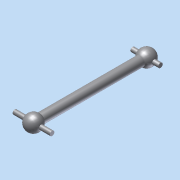
# Autodesk Inventor part: Tie Rod
Saved by Autodesk Inventor 2011 SP1 (Build 150282100, 282)
## iProperties
Created: 2011-09-20
Part Number: Tie Rod
Document SubType Name: Modeling
Designer: dgitz
Density: 1 g/cm^3
Author: dgitz
Autodesk Inventor part; units mm, degrees
ref_plane "XZ Plane" through (0, 0, 0) normal (0, 1, 0) x (-1, 0, 0)
sketch "Sketch1" plane through (0, 0, 0) normal (0, 0, 1) x (1, 0, 0)
  circle A0 centre (0, 0) radius 2.032
  dimension "d0" = 4.064
  constraints: 1 centre point, 1 coincident
  measures "d0" diameter of A0
extrude "Extrusion1" add sketch "Sketch1" along normal mid plane 42.926
sketch "Sketch2" plane through (0, 0, 0) normal (0, 1, 0) x (-1, 0, 0)
  arc A0 (2.032, 21.463) -> (0, 27.6541) centre (0, 24.2251) ccw
  line L0 (0, 21.463) -> (2.032, 21.463)
  line L1 (2.032, -21.463) -> (-2.032, -21.463) projected
  line L2 (-2.032, -21.463) -> (-2.032, 21.463) projected
  line L3 (-2.032, 21.463) -> (2.032, 21.463) projected
  line L4 (2.032, 21.463) -> (2.032, -21.463) projected
  line L5 (12.7779, 0) -> (0, 0) construction
  arc A1 (-2.032, -21.463) -> (0, -27.6541) centre (0, -24.2251) ccw
  line L6 (-2.032, -21.463) -> (0, -21.463)
  line L7 (0, 21.463) -> (0, 27.6541)
  line L8 (2.032, -21.463) -> (-2.032, -21.463) projected
  line L9 (0, -27.6541) -> (0, -21.463)
  point P0 (0, -24.5585)
  dimension "d3" = 6.858
  constraints: 10 end point, 4 point on circle, 2 centre point, 2 horizontal, 2 midpoint, 2 symmetric about line, 2 vertical, 1 point on line, 1 other
  measures "d3" diameter of A0
revolve "Revolution1" add sketch "Sketch2" angle 360 about axis through (0, 0, 21.463) along (0, 0, 1) contours L0 L7 A0 | L9 A1 L1
ref_plane "Work Plane1" through (8.001, 0, 0) normal (1, 0, 0) x (0, 1, 0)
sketch "Sketch3" plane through (8.001, 0, 0) normal (1, 0, 0) x (0, 1, 0)
  circle A0 centre (0, 24.2251) radius 0.9525
  arc A1 (2.032, 21.463) -> (-2.032, 21.463) centre (0, 24.2251) ccw projected
  point P0 (0, 0)
  dimension "d6" = 1.905
  constraints: 1 centre point, 1 concentric
  measures "d6" diameter of A0
extrude "Extrusion2" add sketch "Sketch3" against normal up to surface
mirror "Mirror1" about plane through (0, 0, 0) normal (1, 0, 0) of "Extrusion2"
ref_plane "Work Plane2" through (5.969, 0, 0) normal (1, 0, 0) x (0, 1, 0)
sketch "Sketch4" plane through (5.969, 0, 0) normal (1, 0, 0) x (0, 1, 0)
  circle A0 centre (0, -24.2251) radius 0.9525
  circle A1 centre (0, 24.2251) radius 0.9525 projected
  arc A2 (-2.032, -21.463) -> (2.032, -21.463) centre (0, -24.2251) ccw projected
  point P0 (0, 0)
  dimension "d10" = 1.905
  constraints: 1 centre point, 1 concentric
  measures "d10" diameter of A0
extrude "Extrusion3" add sketch "Sketch4" against normal up to surface contours A0
mirror "Mirror2" about plane through (0, 0, 0) normal (1, 0, 0) of "Extrusion3"
body "Solid1"
